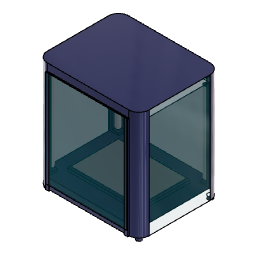
UV 2 FULL v4 (Autodesk Fusion 360 design; units mm, degrees)
Autodesk Fusion 360 part; units mm, degrees
sketch "Sketch1" plane through (0, 0, 0) normal (0, 0, 1) x (1, 0, 0)
  line L0 (40, 40) -> (-40, 40)
  line L1 (-50, 30) -> (-50, -30)
  line L2 (-40, -40) -> (40, -40)
  line L3 (50, -30) -> (50, 30)
  line L4 (50, 40) -> (-50, -40) construction
  line L5 (-50, 40) -> (50, -40) construction
  arc A0 (-40, 40) -> (-50, 30) centre (-40, 30) ccw
  arc A1 (50, 30) -> (40, 40) centre (40, 30) ccw
  arc A2 (40, -40) -> (50, -30) centre (40, -30) ccw
  arc A3 (-50, -30) -> (-40, -40) centre (-40, -30) ccw
  dimension "d1" = 100
  dimension "d2" = 80
  dimension "d3" = 10
  dimension "d4" = 10
  constraint horizontal L0
  constraint perpendicular L0 L1
  constraint parallel L0 L2
  constraint parallel L1 L3
  constraint coincident L4 origin
  constraint coincident L5 origin
  constraint coincident L5.start L0
  constraint coincident L5.start L1
  constraint tangent L0 A0
  constraint tangent L1 A0
  constraint coincident L4.start L3
  constraint coincident L4.start L0
  constraint tangent L3 A1
  constraint tangent L0 A1
  constraint coincident L5.end L3
  constraint coincident L5.end L2
  constraint tangent L3 A2
  constraint tangent L2 A2
  constraint equal A1 A2
  constraint coincident L4.end L1
  constraint coincident L4.end L2
  constraint tangent L1 A3
  constraint tangent L2 A3
  constraint equal A1 A3
  measures "d1" distance of L4.end L5.end
  measures "d2" distance of L5.start L4.end
  measures "d3" radius of A0
  measures "d4" radius of A1
extrude "Extrude1" add sketch "Sketch1" along normal blind 12 makes body 1
sketch "Sketch2" plane through (0, 0, 12) normal (0, 0, 1) x (-1, 0, 0)
  arc A0 (50, 30) -> (40, 40) centre (40, 30) ccw
  line L0 (40, 40) -> (-40, 40)
  arc A1 (-40, 40) -> (-50, 30) centre (-40, 30) ccw
  line L1 (-50, 30) -> (-50, -30)
  arc A2 (-50, -30) -> (-40, -40) centre (-40, -30) ccw
  line L2 (-40, -40) -> (40, -40)
  arc A3 (40, -40) -> (50, -30) centre (40, -30) ccw
  line L3 (50, -30) -> (50, 30)
  line L4 (46.5, -30) -> (46.5, 30)
  arc A4 (46.5, 30) -> (40, 36.5) centre (40, 30) ccw
  line L5 (40, 36.5) -> (-40, 36.5)
  arc A5 (-40, 36.5) -> (-46.5, 30) centre (-40, 30) ccw
  line L6 (-46.5, 30) -> (-46.5, -30)
  arc A6 (-46.5, -30) -> (-40, -36.5) centre (-40, -30) ccw
  line L7 (-40, -36.5) -> (40, -36.5)
  arc A7 (40, -36.5) -> (46.5, -30) centre (40, -30) ccw
  dimension "d7" = -3.5
extrude "Extrude2" add sketch "Sketch2" along normal blind 95 bodies 1
sketch "Sketch3" plane through (50, 0, 0) normal (1, 0, 0) x (0, 1, 0)
  line L0 (-30, 0) -> (30, 0)
  line L1 (30, 0) -> (30, 107)
  line L2 (30, 107) -> (-30, 107)
  line L3 (-30, 107) -> (-30, 0)
  line L4 (-30, 100) -> (30, 100)
  line L5 (30, 100) -> (30, 10)
  line L6 (30, 10) -> (-30, 10)
  line L7 (-30, 10) -> (-30, 100)
  dimension "d10" = 60
  dimension "d11" = 90
  constraint horizontal L4
  constraint vertical L5
  constraint horizontal L6
  constraint vertical L7
  constraint coincident L3 L4.start
  measures "d10" distance of L4.start L4.end
  measures "d11" distance of L4.start L6.end
extrude "Extrude3" cut sketch "Sketch3" against normal blind 170 contours L1 L3 L4 L5 L6 L7 bodies 1
sketch "Sketch4" plane through (0, -40, 0) normal (0, -1, 0) x (1, 0, 0)
  line L0 (-40, 0) -> (40, 0)
  line L1 (40, 0) -> (40, 107)
  line L2 (40, 107) -> (-40, 107)
  line L3 (-40, 107) -> (-40, 0)
  line L4 (-40, 100) -> (40, 100)
  line L5 (40, 100) -> (40, 10)
  line L6 (40, 10) -> (-40, 10)
  line L7 (-40, 10) -> (-40, 100)
  dimension "d14" = 80
  dimension "d15" = 90
  constraint horizontal L4
  constraint vertical L5
  constraint horizontal L6
  constraint vertical L7
  constraint coincident L3 L4.start
  measures "d14" distance of L4.start L4.end
  measures "d15" distance of L4.start L6.end
extrude "Extrude4" cut sketch "Sketch4" against normal blind 135 contours L1 L3 L4 L5 L6 L7 bodies 1
sketch "Sketch5" plane through (0, 0, 10) normal (0, 0, 1) x (-1, 0, 0)
  line L0 (-40, 30) -> (-50, 30)
  line L1 (-50, 30) -> (-50, -30)
  line L2 (-50, -30) -> (-40, -30)
  line L3 (-40, -30) -> (-40, -40)
  line L4 (-40, -40) -> (40, -40)
  line L5 (40, -40) -> (40, -30)
  line L6 (40, -30) -> (50, -30)
  line L7 (50, -30) -> (50, 30)
  line L8 (50, 30) -> (40, 30)
  line L9 (40, 30) -> (40, 40)
  line L10 (40, 40) -> (-40, 40)
  line L11 (-40, 40) -> (-40, 30)
  line L12 (35, -25) -> (-35, -25)
  line L13 (-35, -25) -> (-35, 25)
  line L14 (-35, 25) -> (35, 25)
  line L15 (35, 25) -> (35, -25)
  dimension "d18" = 70
  dimension "d19" = 50
  constraint horizontal L12
  constraint vertical L13
  constraint horizontal L14
  constraint vertical L15
  measures "d18" distance of L12.start L12.end
  measures "d19" distance of L12.start L14.end
extrude "Extrude5" add sketch "Sketch5" along normal blind 4 contours L12 L13 L14 L15 bodies 1
fillet "Fillet1" radius 1.5 1 faces at (-11.6667, 8.3333, 14) on bodies 1
cylinder "CylinderPrimitive1" add diameter 4.8 height 80 placed x (1, 0, 0) y (0, 1, 0) z (0, 0, 1) at (43.2293, -32.75, 14) bodies 1
mirror "Mirror1" about plane through (0, 0, 0) normal (1, 0, 0) of "CylinderPrimitive1"
mirror "Mirror2" about plane through (0, 0, 0) normal (0, 1, 0) of "CylinderPrimitive1", "Mirror1"
sketch "Sketch7" plane through (50, 0, 0) normal (1, 0, 0) x (0, 1, 0)
  line L0 (-30, 100) -> (30, 100)
  line L1 (30, 100) -> (30, 107)
  line L2 (30, 107) -> (-30, 107)
  line L3 (-30, 107) -> (-30, 100)
  line L4 (-30, 100) -> (30, 100)
  line L5 (30, 100) -> (30, 10)
  line L6 (30, 10) -> (-30, 10)
  line L7 (-30, 10) -> (-30, 100)
  constraint horizontal L4
  constraint vertical L5
  constraint horizontal L6
  constraint vertical L7
  constraint coincident L0.start L3.end
sketch "Sketch8" plane through (0, 40, 0) normal (0, 1, 0) x (-1, 0, 0)
  line L0 (-40, 100) -> (40, 100)
  line L1 (40, 100) -> (40, 107)
  line L2 (40, 107) -> (-40, 107)
  line L3 (-40, 107) -> (-40, 100)
  line L4 (-40, 100) -> (40, 100)
  line L5 (40, 100) -> (40, 10)
  line L6 (40, 10) -> (-40, 10)
  line L7 (-40, 10) -> (-40, 100)
  constraint horizontal L4
  constraint vertical L5
  constraint horizontal L6
  constraint vertical L7
  constraint coincident L0.start L3.end
sketch "Sketch9" plane through (-50, 0, 0) normal (-1, 0, 0) x (0, -1, 0)
  line L0 (-30, 100) -> (30, 100)
  line L1 (30, 100) -> (30, 107)
  line L2 (30, 107) -> (-30, 107)
  line L3 (-30, 107) -> (-30, 100)
  line L4 (-30, 100) -> (30, 100)
  line L5 (30, 100) -> (30, 10)
  line L6 (30, 10) -> (-30, 10)
  line L7 (-30, 10) -> (-30, 100)
  constraint horizontal L4
  constraint vertical L5
  constraint horizontal L6
  constraint vertical L7
  constraint coincident L0.start L3.end
extrude "Extrude6" add sketch "Sketch9" against normal blind 1 contours L0 L4 L5 L6 L7 bodies 1
extrude "Extrude7" add sketch "Sketch8" against normal blind 1 contours L0 L4 L5 L6 L7 bodies 1
extrude "Extrude8" add sketch "Sketch7" against normal blind 1 contours L0 L4 L5 L6 L7 bodies 1
sketch "Sketch10" plane through (0, 0, 107) normal (0, 0, 1) x (-1, 0, 0)
  arc A0 (40, -36.5) -> (46.5, -30) centre (40, -30) ccw
  line L0 (40, -36.5) -> (-40, -36.5)
  arc A1 (-46.5, -30) -> (-40, -36.5) centre (-40, -30) ccw
  line L1 (-46.5, -30) -> (-46.5, 30)
  arc A2 (-40, 36.5) -> (-46.5, 30) centre (-40, 30) ccw
  line L2 (-40, 36.5) -> (40, 36.5)
  arc A3 (46.5, 30) -> (40, 36.5) centre (40, 30) ccw
  line L3 (46.5, 30) -> (46.5, -30)
  line L4 (50, -30) -> (50, 30)
  arc A4 (50, 30) -> (40, 40) centre (40, 30) ccw
  line L5 (40, 40) -> (-40, 40)
  arc A5 (-40, 40) -> (-50, 30) centre (-40, 30) ccw
  line L6 (-50, 30) -> (-50, -30)
  arc A6 (-50, -30) -> (-40, -40) centre (-40, -30) ccw
  line L7 (-40, -40) -> (40, -40)
  arc A7 (40, -40) -> (50, -30) centre (40, -30) ccw
  line L8 (49.0553, -30) -> (49.0553, 30)
  arc A8 (49.0553, 30) -> (40, 39.0553) centre (40, 30) ccw
  line L9 (40, 39.0553) -> (-40, 39.0553)
  arc A9 (-40, 39.0553) -> (-49.0553, 30) centre (-40, 30) ccw
  line L10 (-49.0553, 30) -> (-49.0553, -30)
  arc A10 (-49.0553, -30) -> (-40, -39.0553) centre (-40, -30) ccw
  line L11 (-40, -39.0553) -> (40, -39.0553)
  arc A11 (40, -39.0553) -> (49.0553, -30) centre (40, -30) ccw
  dimension "d36" = -0.9447
extrude "Extrude9" add sketch "Sketch10" against normal blind 5 contours A0 L0 A1 L1 A2 L2 A3 L3 bodies 1
sketch "Sketch11" plane through (-50, 0, 0) normal (-1, 0, 0) x (0, -1, 0)
  line L0 (30, 0) -> (30, 107)
  line L1 (30, 107) -> (-30, 107)
  line L2 (-30, 107) -> (-30, 0)
  line L3 (-30, 0) -> (30, 0)
  line L4 (-30, 100) -> (30, 100)
  line L5 (-30, 100) -> (-30, 107)
  line L6 (30, 107) -> (30, 100)
  line L7 (30, 107) -> (-30, 107)
  constraint coincident L2 L4.start
  constraint coincident L0 L4.end
  constraint perpendicular L0 L4
  constraint coincident L1.end L2.start
  constraint coincident L0.end L1.start
extrude "Extrude10" add sketch "Sketch11" against normal blind 100 contours L0 L1 L2 L4 L5 L6 L7 bodies 1
sketch "Sketch12" plane through (0, 0, 0) normal (0, 0, -1) x (1, 0, 0)
  arc A0 (-40, 40) -> (-50, 30) centre (-40, 30) ccw
  line L0 (-50, 30) -> (-50, -30)
  arc A1 (-50, -30) -> (-40, -40) centre (-40, -30) ccw
  line L1 (-40, -40) -> (40, -40)
  arc A2 (40, -40) -> (50, -30) centre (40, -30) ccw
  line L2 (50, -30) -> (50, 30)
  arc A3 (50, 30) -> (40, 40) centre (40, 30) ccw
  line L3 (40, 40) -> (-40, 40)
  line L4 (-40, 40) -> (-40, 41)
  line L5 (-40, 41) -> (-37, 41)
  line L6 (-37, 41) -> (-37, 41.5)
  line L7 (-37, 41.5) -> (-40.5, 41.5)
  line L8 (-40.5, 41.5) -> (-40.5, 39.9875)
  line L9 (-40.5, 39.9875) -> (-40, 40)
  line L10 (0, 54) -> (0, 19) construction
  line L11 (37, 41.5) -> (40.5, 41.5)
  line L12 (40.5, 41.5) -> (40.5, 39.9875)
  line L13 (40, 40) -> (40, 41)
  line L14 (40, 41) -> (37, 41)
  line L15 (37, 41) -> (37, 41.5)
  line L16 (40.5, 39.9875) -> (40, 40)
  constraint coincident A0.start L3.end
  constraint perpendicular L3 L4
  constraint perpendicular L4 L5
  constraint perpendicular L5 L6
  constraint perpendicular L4 L7
  constraint coincident A0 L8.end
  constraint perpendicular L7 L8
  constraint perpendicular L3 L10
  constraint symmetric A0.start L10 A3.end
  constraint symmetric L4.end L10 L13.end
  constraint symmetric L5.end L10 L14.end
  constraint symmetric L6.end L10 L11.start
  constraint symmetric L7.end L10 L11.end
  constraint symmetric L8.end L10 L12.end
extrude "Extrude11" add sketch "Sketch12" against normal blind 100 contours A0 L4 L5 L6 L7 L8 | A3 L11 L12 L13 L14 L15 bodies 1
sketch "Sketch13" plane through (0, 0, 100) normal (0, 0, 1) x (-1, 0, 0)
  line L0 (40, 41) -> (40, 40)
  arc A0 (40.5, 39.9875) -> (40, 40) centre (40, 30) ccw
  line L1 (40.5, 39.9875) -> (40.5, 41.5)
  line L2 (40.5, 41.5) -> (37, 41.5)
  line L3 (37, 41.5) -> (37, 41)
  line L4 (37, 41) -> (40, 41)
  line L5 (40, 41) -> (-40, 41)
  line L6 (-40, 41) -> (-40, 40)
  line L7 (-40, 40) -> (40, 40)
  line L8 (40, 40) -> (40, 41)
  constraint horizontal L5
  constraint vertical L6
  constraint horizontal L7
  constraint vertical L8
  constraint coincident L0.start L4.end
extrude "Extrude1'" add sketch "Sketch13" against normal blind 95 separate body contours L0 L4 L5 L6 L7 L8 makes body 2 in component "Component"
sketch "Sketch14" plane through (0, 0, 0) normal (0, 0, -1) x (1, 0, 0)
  arc A0 (-40.5, 39.9875) -> (-50, 30) centre (-40, 30) ccw
  line L0 (-50, 30) -> (-50, -30)
  arc A1 (-50, -30) -> (-40, -40) centre (-40, -30) ccw
  line L1 (-40, -40) -> (40, -40)
  arc A2 (40, -40) -> (50, -30) centre (40, -30) ccw
  line L2 (50, -30) -> (50, 30)
  arc A3 (50, 30) -> (40.5, 39.9875) centre (40, 30) ccw
  line L3 (40.5, 39.9875) -> (40.5, 41.5)
  line L4 (40.5, 41.5) -> (37, 41.5)
  line L5 (37, 41.5) -> (37, 41)
  line L6 (37, 41) -> (40, 41)
  line L7 (40, 41) -> (40, 40)
  line L8 (40, 40) -> (-40, 40)
  line L9 (-40, 40) -> (-40, 41)
  line L10 (-40, 41) -> (-37, 41)
  line L11 (-37, 41) -> (-37, 41.5)
  line L12 (-37, 41.5) -> (-40.5, 41.5)
  line L13 (-40.5, 41.5) -> (-40.5, 39.9875)
  circle A4 centre (-45, 35) radius 2.5
  circle A5 centre (45, 35) radius 2.5
  circle A6 centre (-45, -35) radius 2.5
  circle A7 centre (45, -35) radius 2.5
  dimension "d51" = 5
  dimension "d52" = 5
  dimension "d53" = 5
  dimension "d54" = 5
  measures "d51" diameter of A4
  measures "d52" diameter of A5
  measures "d53" diameter of A6
  measures "d54" diameter of A7
extrude "Extrude12" add sketch "Sketch14" along normal blind 3 contours A4 | A5 | A6 | A7 bodies 1
component "Component" placed x (1, 0, 0) y (0, 1, 0) z (0, 0, 1) at (-0.5, -0.5, 0)
